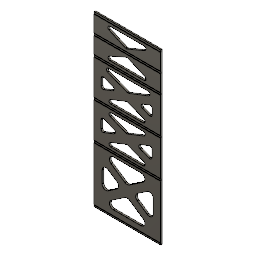
ShelfBack v12 (Autodesk Fusion 360 design; units mm, degrees)
Autodesk Fusion 360 part; units mm, degrees
sketch "Sketch1" plane through (0, 0, 0) normal (0, 0, 1) x (1, 0, 0)
  line L0 (0, 0) -> (457.2, 0)
  line L1 (457.2, 0) -> (457.2, 1155.7)
  line L2 (457.2, 1155.7) -> (0, 1155.7)
  line L3 (0, 1155.7) -> (0, 0)
  line L4 (133.4674, 50.8) -> (323.7326, 50.8)
  line L5 (133.4674, 361.95) -> (323.7326, 361.95)
  line L6 (119.2053, 315.5321) -> (214.3379, 250.9779)
  line L7 (242.8621, 250.9779) -> (337.9947, 315.5321)
  line L8 (119.2053, 97.2179) -> (214.3379, 161.7721)
  line L9 (242.8621, 161.7721) -> (337.9947, 97.2179)
  line L10 (406.4, 252.627) -> (406.4, 160.123)
  line L11 (366.7379, 273.6449) -> (298.577, 227.3929)
  line L12 (298.577, 185.3571) -> (366.7379, 139.1051)
  line L13 (58.3986, 247.4708) -> (58.3986, 165.2792)
  line L14 (98.0607, 268.4887) -> (158.623, 227.3929)
  line L15 (158.623, 185.3571) -> (98.0607, 144.2613)
  arc A0 (98.0607, 268.4887) -> (58.3986, 247.4708) centre (83.7986, 247.4708) ccw
  arc A1 (58.3986, 165.2792) -> (98.0607, 144.2613) centre (83.7986, 165.2792) ccw
  arc A2 (158.623, 185.3571) -> (158.623, 227.3929) centre (144.3608, 206.375) ccw
  arc A3 (298.577, 227.3929) -> (298.577, 185.3571) centre (312.8392, 206.375) ccw
  arc A4 (406.4, 252.627) -> (366.7379, 273.6449) centre (381, 252.627) ccw
  arc A5 (366.7379, 139.1051) -> (406.4, 160.123) centre (381, 160.123) ccw
  arc A6 (337.9947, 315.5321) -> (323.7326, 361.95) centre (323.7326, 336.55) ccw
  arc A7 (133.4674, 361.95) -> (119.2053, 315.5321) centre (133.4674, 336.55) ccw
  arc A8 (214.3379, 250.9779) -> (242.8621, 250.9779) centre (228.6, 271.9958) ccw
  arc A9 (119.2053, 97.2179) -> (133.4674, 50.8) centre (133.4674, 76.2) ccw
  arc A10 (323.7326, 50.8) -> (337.9947, 97.2179) centre (323.7326, 76.2) ccw
  arc A11 (242.8621, 161.7721) -> (214.3379, 161.7721) centre (228.6, 140.7542) ccw
  line L16 (117.8597, 412.75) -> (339.3403, 412.75)
  line L17 (117.8597, 615.95) -> (339.3403, 615.95)
  line L18 (113.2159, 591.4295) -> (223.9562, 547.9243)
  line L19 (233.2438, 547.9243) -> (343.9841, 591.4295)
  line L20 (113.2159, 437.2705) -> (223.9562, 480.7757)
  line L21 (233.2438, 480.7757) -> (343.9841, 437.2705)
  line L22 (397.7814, 539.3504) -> (397.7814, 489.3496)
  line L23 (380.4376, 551.1709) -> (316.8002, 526.1705)
  line L24 (316.8002, 502.5295) -> (380.4376, 477.5291)
  line L25 (50.8, 542.7363) -> (50.8, 485.9637)
  line L26 (68.1438, 554.5568) -> (140.3998, 526.1705)
  line L27 (140.3998, 502.5295) -> (68.1438, 474.1432)
  arc A12 (223.9562, 547.9243) -> (233.2438, 547.9243) centre (228.6, 559.7449) ccw
  arc A13 (223.9562, 547.9243) -> (233.2438, 547.9243) centre (228.6, 559.7449) ccw
  arc A14 (117.8597, 615.95) -> (113.2159, 591.4295) centre (117.8597, 603.25) ccw
  arc A15 (343.9841, 591.4295) -> (339.3403, 615.95) centre (339.3403, 603.25) ccw
  arc A16 (316.8002, 526.1705) -> (316.8002, 502.5295) centre (321.444, 514.35) ccw
  arc A17 (397.7814, 539.3504) -> (380.4376, 551.1709) centre (385.0814, 539.3504) ccw
  arc A18 (380.4376, 477.5291) -> (397.7814, 489.3496) centre (385.0814, 489.3496) ccw
  arc A19 (68.1438, 554.5568) -> (50.8, 542.7363) centre (63.5, 542.7363) ccw
  arc A20 (50.8, 485.9637) -> (68.1438, 474.1432) centre (63.5, 485.9637) ccw
  arc A21 (140.3998, 502.5295) -> (140.3998, 526.1705) centre (135.756, 514.35) ccw
  arc A22 (233.2438, 480.7757) -> (223.9562, 480.7757) centre (228.6, 468.9551) ccw
  arc A23 (113.2159, 437.2705) -> (117.8597, 412.75) centre (117.8597, 425.45) ccw
  arc A24 (339.3403, 412.75) -> (343.9841, 437.2705) centre (339.3403, 425.45) ccw
  arc A25 (339.3403, 666.75) -> (343.9841, 691.2705) centre (339.3403, 679.45) ccw
  line L28 (240.8287, 792.2041) -> (376.3113, 845.4295)
  line L29 (399.6698, 781.3923) -> (399.6698, 742.6077)
  line L30 (382.3261, 793.2128) -> (332.9639, 773.8205)
  line L31 (113.2159, 691.2705) -> (223.9562, 734.7757)
  arc A26 (382.3261, 730.7872) -> (399.6698, 742.6077) centre (386.9698, 742.6077) ccw
  arc A27 (113.2159, 691.2705) -> (117.8597, 666.75) centre (117.8597, 679.45) ccw
  arc A28 (332.9639, 773.8205) -> (332.9639, 750.1795) centre (337.6077, 762) ccw
  line L32 (332.9639, 750.1795) -> (382.3261, 730.7872)
  arc A29 (399.6698, 781.3923) -> (382.3261, 793.2128) centre (386.9698, 781.3923) ccw
  line L33 (233.2438, 734.7757) -> (343.9841, 691.2705)
  arc A30 (376.3113, 845.4295) -> (371.6676, 869.95) centre (371.6676, 857.25) ccw
  line L34 (117.8597, 666.75) -> (339.3403, 666.75)
  line L35 (69.0988, 801.4412) -> (131.821, 776.8003)
  arc A31 (233.2438, 734.7757) -> (223.9562, 734.7757) centre (228.6, 722.9551) ccw
  line L36 (96.0585, 845.4295) -> (231.5411, 792.2041)
  line L37 (131.821, 753.1592) -> (69.0988, 728.5184)
  line L38 (51.755, 789.6207) -> (51.755, 740.3389)
  arc A32 (51.755, 740.3389) -> (69.0988, 728.5184) centre (64.455, 740.3389) ccw
  line L39 (100.7023, 869.95) -> (371.6676, 869.95)
  arc A33 (69.0988, 801.4412) -> (51.755, 789.6207) centre (64.455, 789.6207) ccw
  arc A34 (131.821, 753.1592) -> (131.821, 776.8003) centre (127.1772, 764.9798) ccw
  arc A35 (231.5411, 792.2041) -> (240.8287, 792.2041) centre (236.1849, 804.0247) ccw
  arc A36 (231.5411, 792.2041) -> (240.8287, 792.2041) centre (236.1849, 804.0247) ccw
  arc A37 (100.7023, 869.95) -> (96.0585, 845.4295) centre (100.7023, 857.25) ccw
  line L40 (111.8118, 920.75) -> (345.3547, 920.75)
  line L41 (106.7442, 945.0951) -> (223.4808, 995.8951)
  line L42 (233.6134, 995.8963) -> (350.4197, 945.0963)
  arc A38 (233.6134, 995.8963) -> (223.4808, 995.8951) centre (228.5484, 984.25) ccw
  arc A39 (345.3547, 920.75) -> (350.4197, 945.0963) centre (345.3547, 933.45) ccw
  arc A40 (106.7442, 945.0951) -> (111.8118, 920.75) centre (111.8118, 933.45) ccw
  line L43 (343.8055, 1123.95) -> (110.2649, 1123.95)
  line L44 (-48.7007, 12.7) -> (-23.0919, 12.7)
  line L45 (-51.4599, 381) -> (-22.1394, 381)
  line L46 (-53.3516, 393.7) -> (-21.1936, 393.7)
  line L47 (-54.802, 635) -> (-24.3434, 635)
  line L48 (-53.5836, 647.7) -> (-25.5617, 647.7)
  line L49 (-59.6754, 889) -> (-30.4351, 889)
  line L50 (-57.2387, 901.7) -> (-30.4351, 901.7)
  line L51 (-56.0203, 1016) -> (-26.7801, 1016)
  line L52 (-53.5836, 1028.7) -> (-26.7801, 1028.7)
  line L53 (-60.8937, 1143) -> (-21.9067, 1143)
  line L54 (105.0768, 1099.658) -> (218.5818, 1048.858)
  line L55 (228.7196, 1048.7543) -> (348.7552, 1099.5543)
  arc A41 (110.2649, 1123.95) -> (105.0768, 1099.658) centre (110.2649, 1111.25) ccw
  arc A42 (348.7552, 1099.5543) -> (343.8055, 1123.95) centre (343.8055, 1111.25) ccw
  arc A43 (218.5818, 1048.858) -> (228.7196, 1048.7543) centre (223.7699, 1060.45) ccw
  point P0 (50.8, 50.8)
  point P1 (406.4, 50.8)
  point P2 (50.8, 361.95)
  point P3 (406.4, 361.95)
  point P4 (228.6, 241.3)
  point P5 (228.6, 171.45)
  point P6 (406.4, 300.5585)
  point P7 (406.4, 112.1915)
  point P8 (267.6033, 206.375)
  point P9 (58.3986, 295.4023)
  point P10 (58.3986, 117.3477)
  point P11 (189.5967, 206.375)
  point P12 (50.8, 412.75)
  point P13 (406.4, 412.75)
  point P14 (50.8, 615.95)
  point P15 (406.4, 615.95)
  point P16 (228.6, 546.1)
  point P17 (228.6, 495.3)
  point P18 (397.7814, 557.9846)
  point P19 (397.7814, 470.7154)
  point P20 (286.7116, 514.35)
  point P21 (50.8, 561.3704)
  point P22 (50.8, 467.3296)
  point P23 (170.4884, 514.35)
  point P24 (228.6, 749.3)
  point P25 (51.755, 808.2548)
  point P26 (406.4, 666.75)
  point P27 (50.8, 666.75)
  point P28 (228.6, 800.1)
  point P29 (33.6425, 869.95)
  point P30 (438.7273, 869.95)
  point P31 (302.8752, 762)
  point P32 (399.6698, 800.0265)
  point P33 (399.6698, 723.9735)
  point P34 (51.755, 721.7047)
  point P35 (161.9097, 764.9798)
  point P36 (50.8, 920.75)
  point P37 (406.4, 920.75)
  point P38 (228.6, 984.25)
  point P39 (406.4, 1123.95)
  point P40 (50.8, 1123.95)
  point P41 (224.3285, 1060.45)
  dimension "d1" = 1155.7
  dimension "d2" = 457.2
  dimension "d14" = 50.8
  dimension "d15" = 50.8
  dimension "d16" = 50.8
  dimension "d18" = 50.8
  dimension "d19" = 50.8
  dimension "d20" = 120.65
  dimension "d21" = 228.6
  dimension "d22" = 228.6
  dimension "d23" = 120.65
  dimension "d24" = 50.8
  dimension "d25" = 50.8
  dimension "d26" = 50.8
  dimension "d27" = 50.8
  dimension "d28" = 50.8
  dimension "d29" = 50.8
  dimension "d30" = 50.8
  dimension "d31" = 50.8
  dimension "d32" = 50.8
  dimension "d33" = 25.4
  dimension "d35" = 50.8
  dimension "d36" = 50.8
  dimension "d38" = 50.8
  dimension "d39" = 50.8
  dimension "d40" = 69.85
  dimension "d41" = 50.8
  dimension "d42" = 50.8
  dimension "d43" = 50.8
  dimension "d44" = 50.8
  dimension "d45" = 50.8
  dimension "d46" = 50.8
  dimension "d47" = 50.8
  dimension "d48" = 50.8
  dimension "d49" = 50.8
  dimension "d50" = 50.8
  dimension "d51" = 12.7
  dimension "d52" = 12.7
  dimension "d53" = 12.7
  dimension "d54" = 12.7
  dimension "d55" = 12.7
  dimension "d56" = 12.7
  dimension "d58" = 69.85
  dimension "d59" = 50.8
  dimension "d60" = 50.8
  dimension "d61" = 50.8
  dimension "d62" = 50.8
  dimension "d63" = 50.8
  dimension "d64" = 50.8
  dimension "d65" = 50.8
  dimension "d66" = 50.8
  dimension "d67" = 50.8
  dimension "d68" = 12.7
  dimension "d69" = 12.7
  dimension "d70" = 12.7
  dimension "d71" = 12.7
  dimension "d72" = 12.7
  dimension "d73" = 12.7
  dimension "d74" = 50.8
  dimension "d75" = 50.8
  dimension "d77" = 12.7
  dimension "d78" = 12.7
  dimension "d79" = 12.7
  dimension "d80" = 50.8
  dimension "d81" = 50.8
  dimension "d84" = 12.7
  dimension "d85" = 368.3
  dimension "d86" = 12.7
  dimension "d89" = 19.05
  dimension "d91" = 50.8
  dimension "d92" = 241.3
  dimension "d93" = 12.7
  dimension "d95" = 19.05
  dimension "d96" = 50.8
  dimension "d97" = 241.3
  dimension "d98" = 12.7
  dimension "d99" = 50.8
  dimension "d100" = 19.05
  dimension "d101" = 114.3
  dimension "d102" = 12.7
  dimension "d103" = 114.3
  dimension "d104" = 19.05
  dimension "d105" = 19.05
  dimension "d107" = 12.7
  dimension "d108" = 12.7
  dimension "d109" = 12.7
  dimension "d110" = 31.75
  dimension "d111" = 31.75
  measures "d1" distance of L0.start L2.end
  measures "d2" distance of L0.start L0.end
  measures "d14" distance of L3 P0
  measures "d15" distance of L0 L4
  measures "d16" distance of L1 P1
  measures "d18" distance of L3 P2
  measures "d19" distance of L1 P3
  measures "d20" distance of L5 P4
  measures "d21" distance of L3 P4
  measures "d22" distance of L3 P5
  measures "d23" distance of L4 P5
  measures "d24" distance of L1 L10
  measures "d25" distance of L7 P6
  measures "d26" distance of L9 P7
  measures "d27" distance of L9 P8
  measures "d28" distance of L7 P8
  measures "d29" distance of L8 P10
  measures "d30" distance of L6 P9
  measures "d31" distance of L6 P11
  measures "d32" distance of L8 P11
  measures "d33" radius of A0
  measures "d35" distance of L3 P12
  measures "d36" distance of L1 P13
  measures "d38" distance of L3 P14
  measures "d39" distance of L1 P15
  measures "d40" distance of L17 P16
  measures "d41" distance of P16 P17
  measures "d42" distance of L19 P18
  measures "d43" distance of L21 P19
  measures "d44" distance of L19 P20
  measures "d45" distance of L21 P20
  measures "d46" distance of L3 L25
  measures "d47" distance of L18 P21
  measures "d48" distance of L20 P22
  measures "d49" distance of L18 P23
  measures "d50" distance of L20 P23
  measures "d51" radius of A12
  measures "d52" radius of A13
  measures "d53" radius of A14
  measures "d54" radius of A16
  measures "d55" radius of A19
  measures "d56" radius of A22
  measures "d58" distance of P28 L39
  measures "d59" distance of P24 P28
  measures "d60" distance of P32 L28
  measures "d61" distance of P33 L33
  measures "d62" distance of P31 L28
  measures "d63" distance of P31 L33
  measures "d64" distance of P25 L36
  measures "d65" distance of P34 L31
  measures "d66" distance of P35 L36
  measures "d67" distance of P35 L31
  measures "d68" radius of A35
  measures "d69" radius of A36
  measures "d70" radius of A37
  measures "d71" radius of A28
  measures "d72" radius of A33
  measures "d73" radius of A31
  measures "d74" distance of L3 P36
  measures "d75" distance of L1 P37
  measures "d77" radius of A38
  measures "d78" radius of A39
  measures "d79" radius of A40
  measures "d80" distance of L3 P40
  measures "d81" distance of L1 P39
  measures "d84" distance of L0.start L44
  measures "d85" distance of L44 L45
  measures "d86" distance of L45 L46
  measures "d89" distance of L5 L45.end
  measures "d91" distance of L5 L16
  measures "d92" distance of L46 L47
  measures "d93" distance of L47 L48
  measures "d95" distance of L17 L47
  measures "d96" distance of L17 L34
  measures "d97" distance of L48 L49
  measures "d98" distance of L49 L50
  measures "d99" distance of L39 L40
  measures "d100" distance of L39 L49
  measures "d101" distance of L50 L51
  measures "d102" distance of L51 L52
  measures "d103" distance of L52 L53
  measures "d104" distance of L40 L50
  measures "d105" distance of L43 L53
  measures "d107" radius of A41
  measures "d108" radius of A42
  measures "d109" radius of A43
  measures "d110" distance of A38.centre L51
  measures "d111" distance of L52 A43.centre
extrude "Extrude2" add sketch "Sketch1" along normal blind 12.7
sketch "Sketch2" plane through (0, 0, 12.7) normal (0, 0, 1) x (1, 0, 0)
  arc A0 (117.8597, 615.95) -> (113.2159, 591.4295) centre (117.8597, 603.25) ccw
  line L0 (117.8597, 615.95) -> (339.3403, 615.95)
  arc A1 (343.9841, 591.4295) -> (339.3403, 615.95) centre (339.3403, 603.25) ccw
  line L1 (343.9841, 591.4295) -> (233.2438, 547.9243)
  arc A2 (223.9562, 547.9243) -> (233.2438, 547.9243) centre (228.6, 559.7449) ccw
  line L2 (223.9562, 547.9243) -> (113.2159, 591.4295)
  arc A3 (397.7814, 539.3504) -> (380.4376, 551.1709) centre (385.0814, 539.3504) ccw
  line L3 (397.7814, 539.3504) -> (397.7814, 489.3496)
  arc A4 (380.4376, 477.5291) -> (397.7814, 489.3496) centre (385.0814, 489.3496) ccw
  line L4 (380.4376, 477.5291) -> (316.8002, 502.5295)
  arc A5 (316.8002, 526.1705) -> (316.8002, 502.5295) centre (321.444, 514.35) ccw
  line L5 (316.8002, 526.1705) -> (380.4376, 551.1709)
  arc A6 (399.6698, 781.3923) -> (382.3261, 793.2128) centre (386.9698, 781.3923) ccw
  line L6 (399.6698, 781.3923) -> (399.6698, 742.6077)
  arc A7 (382.3261, 730.7872) -> (399.6698, 742.6077) centre (386.9698, 742.6077) ccw
  line L7 (382.3261, 730.7872) -> (332.9639, 750.1795)
  arc A8 (332.9639, 773.8205) -> (332.9639, 750.1795) centre (337.6077, 762) ccw
  line L8 (332.9639, 773.8205) -> (382.3261, 793.2128)
  arc A9 (133.4674, 361.95) -> (119.2053, 315.5321) centre (133.4674, 336.55) ccw
  line L9 (133.4674, 361.95) -> (323.7326, 361.95)
  arc A10 (337.9947, 315.5321) -> (323.7326, 361.95) centre (323.7326, 336.55) ccw
  line L10 (337.9947, 315.5321) -> (242.8621, 250.9779)
  arc A11 (214.3379, 250.9779) -> (242.8621, 250.9779) centre (228.6, 271.9958) ccw
  line L11 (214.3379, 250.9779) -> (119.2053, 315.5321)
  arc A12 (406.4, 252.627) -> (366.7379, 273.6449) centre (381, 252.627) ccw
  line L12 (406.4, 252.627) -> (406.4, 160.123)
  arc A13 (366.7379, 139.1051) -> (406.4, 160.123) centre (381, 160.123) ccw
  line L13 (366.7379, 139.1051) -> (298.577, 185.3571)
  arc A14 (298.577, 227.3929) -> (298.577, 185.3571) centre (312.8392, 206.375) ccw
  line L14 (298.577, 227.3929) -> (366.7379, 273.6449)
  arc A15 (113.2159, 437.2705) -> (117.8597, 412.75) centre (117.8597, 425.45) ccw
  line L15 (113.2159, 437.2705) -> (223.9562, 480.7757)
  arc A16 (233.2438, 480.7757) -> (223.9562, 480.7757) centre (228.6, 468.9551) ccw
  line L16 (233.2438, 480.7757) -> (343.9841, 437.2705)
  arc A17 (339.3403, 412.75) -> (343.9841, 437.2705) centre (339.3403, 425.45) ccw
  line L17 (339.3403, 412.75) -> (117.8597, 412.75)
  arc A18 (119.2053, 97.2179) -> (133.4674, 50.8) centre (133.4674, 76.2) ccw
  line L18 (119.2053, 97.2179) -> (214.3379, 161.7721)
  arc A19 (242.8621, 161.7721) -> (214.3379, 161.7721) centre (228.6, 140.7542) ccw
  line L19 (242.8621, 161.7721) -> (337.9947, 97.2179)
  arc A20 (323.7326, 50.8) -> (337.9947, 97.2179) centre (323.7326, 76.2) ccw
  line L20 (323.7326, 50.8) -> (133.4674, 50.8)
  arc A21 (68.1438, 554.5568) -> (50.8, 542.7363) centre (63.5, 542.7363) ccw
  line L21 (68.1438, 554.5568) -> (140.3998, 526.1705)
  arc A22 (140.3998, 502.5295) -> (140.3998, 526.1705) centre (135.756, 514.35) ccw
  line L22 (140.3998, 502.5295) -> (68.1438, 474.1432)
  arc A23 (50.8, 485.9637) -> (68.1438, 474.1432) centre (63.5, 485.9637) ccw
  line L23 (50.8, 485.9637) -> (50.8, 542.7363)
  arc A24 (113.2159, 691.2705) -> (117.8597, 666.75) centre (117.8597, 679.45) ccw
  line L24 (113.2159, 691.2705) -> (223.9562, 734.7757)
  arc A25 (233.2438, 734.7757) -> (223.9562, 734.7757) centre (228.6, 722.9551) ccw
  line L25 (233.2438, 734.7757) -> (343.9841, 691.2705)
  arc A26 (339.3403, 666.75) -> (343.9841, 691.2705) centre (339.3403, 679.45) ccw
  line L26 (339.3403, 666.75) -> (117.8597, 666.75)
  arc A27 (98.0607, 268.4887) -> (58.3986, 247.4708) centre (83.7986, 247.4708) ccw
  line L27 (98.0607, 268.4887) -> (158.623, 227.3929)
  arc A28 (158.623, 185.3571) -> (158.623, 227.3929) centre (144.3608, 206.375) ccw
  line L28 (158.623, 185.3571) -> (98.0607, 144.2613)
  arc A29 (58.3986, 165.2792) -> (98.0607, 144.2613) centre (83.7986, 165.2792) ccw
  line L29 (58.3986, 165.2792) -> (58.3986, 247.4708)
  arc A30 (69.0988, 801.4412) -> (51.755, 789.6207) centre (64.455, 789.6207) ccw
  line L30 (69.0988, 801.4412) -> (131.821, 776.8003)
  arc A31 (131.821, 753.1592) -> (131.821, 776.8003) centre (127.1772, 764.9798) ccw
  line L31 (131.821, 753.1592) -> (69.0988, 728.5184)
  arc A32 (51.755, 740.3389) -> (69.0988, 728.5184) centre (64.455, 740.3389) ccw
  line L32 (51.755, 740.3389) -> (51.755, 789.6207)
  arc A33 (100.7023, 869.95) -> (96.0585, 845.4295) centre (100.7023, 857.25) ccw
  line L33 (100.7023, 869.95) -> (371.6676, 869.95)
  arc A34 (376.3113, 845.4295) -> (371.6676, 869.95) centre (371.6676, 857.25) ccw
  line L34 (376.3113, 845.4295) -> (240.8287, 792.2041)
  arc A35 (231.5411, 792.2041) -> (240.8287, 792.2041) centre (236.1849, 804.0247) ccw
  line L35 (231.5411, 792.2041) -> (96.0585, 845.4295)
  arc A36 (233.6134, 995.8963) -> (223.4808, 995.8951) centre (228.5484, 984.25) ccw
  line L36 (233.6134, 995.8963) -> (350.4197, 945.0963)
  arc A37 (345.3547, 920.75) -> (350.4197, 945.0963) centre (345.3547, 933.45) ccw
  line L37 (345.3547, 920.75) -> (111.8118, 920.75)
  arc A38 (106.7442, 945.0951) -> (111.8118, 920.75) centre (111.8118, 933.45) ccw
  line L38 (106.7442, 945.0951) -> (223.4808, 995.8951)
  arc A39 (218.5818, 1048.858) -> (228.7196, 1048.7543) centre (223.7699, 1060.45) ccw
  line L39 (218.5818, 1048.858) -> (105.0768, 1099.658)
  arc A40 (110.2649, 1123.95) -> (105.0768, 1099.658) centre (110.2649, 1111.25) ccw
  line L40 (110.2649, 1123.95) -> (343.8055, 1123.95)
  arc A41 (348.7552, 1099.5543) -> (343.8055, 1123.95) centre (343.8055, 1111.25) ccw
  line L41 (348.7552, 1099.5543) -> (228.7196, 1048.7543)
  line L42 (0, 1155.7) -> (0, 0)
  line L43 (0, 0) -> (457.2, 0)
  line L44 (457.2, 0) -> (457.2, 1155.7)
  line L45 (457.2, 1155.7) -> (0, 1155.7)
  line L46 (0, 1155.7) -> (457.2, 1155.7)
  line L47 (457.2, 1155.7) -> (457.2, 1142.7)
  line L48 (457.2, 1142.7) -> (0, 1142.7)
  line L49 (0, 1142.7) -> (0, 1155.7)
  line L50 (0, 1028.7) -> (457.2, 1028.7)
  line L51 (457.2, 1028.7) -> (457.2, 1015.7)
  line L52 (457.2, 1015.7) -> (0, 1015.7)
  line L53 (0, 1015.7) -> (0, 1028.7)
  line L54 (0, 901.7) -> (457.2, 901.7)
  line L55 (457.2, 901.7) -> (457.2, 888.7)
  line L56 (457.2, 888.7) -> (0, 888.7)
  line L57 (0, 888.7) -> (0, 901.7)
  line L58 (0, 647.7) -> (457.2, 647.7)
  line L59 (457.2, 647.7) -> (457.2, 634.7)
  line L60 (457.2, 634.7) -> (0, 634.7)
  line L61 (0, 634.7) -> (0, 647.7)
  line L62 (0, 393.7) -> (457.2, 393.7)
  line L63 (457.2, 393.7) -> (457.2, 380.7)
  line L64 (457.2, 380.7) -> (0, 380.7)
  line L65 (0, 380.7) -> (0, 393.7)
  line L66 (0, 12.7) -> (457.2, 12.7)
  line L67 (457.2, 12.7) -> (457.2, -0.3)
  line L68 (457.2, -0.3) -> (0, -0.3)
  line L69 (0, -0.3) -> (0, 12.7)
  dimension "d116" = 13
  dimension "d117" = 127
  dimension "d118" = 13
  dimension "d119" = 127
  dimension "d120" = 13
  dimension "d121" = 254
  dimension "d122" = 13
  dimension "d123" = 254
  dimension "d124" = 13
  dimension "d125" = 381
  dimension "d126" = 13
  measures "d116" distance of L44.end L47.end
  measures "d117" distance of L46 L50
  measures "d118" distance of L50.end L51.end
  measures "d119" distance of L50 L54
  measures "d120" distance of L54.end L55.end
  measures "d121" distance of L54 L58
  measures "d122" distance of L58.end L59.end
  measures "d123" distance of L58 L62
  measures "d124" distance of L62.end L63.end
  measures "d125" distance of L62 L66
  measures "d126" distance of L66.end L67.end
extrude "Extrude3" cut sketch "Sketch2" against normal blind 2 contours L42 L44 L45 L46 L47 L48 L49 | L42 L44 L50 L51 L52 L53 | L42 L44 L54 L55 L56 L57 | L42 L44 L58 L59 L60 L61 | L42 L44 L62 L63 L64 L65 | L42 L43 L44 L66 L67 L69
extrude "Extrude1" [suppressed]
equation "d40 = ( 7.5 in - 2 in ) / 2"
equation "d58 = ( 7.5 in - 2 in ) / 2"
